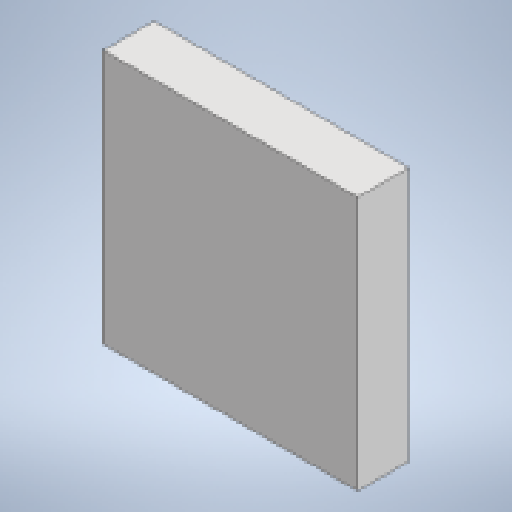
# Autodesk Inventor part: Contrapeso
Saved by Autodesk Inventor 2024 (Build 280153000, 153)
## iProperties
Created: 2024-07-16
Part Number: Contrapeso
Material: Genérico
Document SubType Name: Modeling
Designer: sergi
Density: 1 g/cm^3
Appearance: Valor por defecto
Author: sergi
Autodesk Inventor part; units mm, degrees
ref_plane "YZ Plane" through (0, 0, 0) normal (1, 0, 0) x (0, 1, 0)
ref_plane "XZ Plane" through (0, 0, 0) normal (0, 1, 0) x (-1, 0, 0)
ref_plane "XY Plane" through (0, 0, 0) normal (0, 0, 1) x (1, 0, 0)
sketch "Boceto1" plane through (0, 0, 0) normal (0, 0, 1) x (1, 0, 0)
  line L0 (0, -3) -> (0, -206) projected
  line L1 (0, -3) -> (-3, -3) projected
  line L2 (-3, -206) -> (-3, -3) projected
  line L3 (0, -206) -> (-3, -206) projected
  line L4 (-206, -203) -> (-206, 0) projected
  line L5 (-206, -203) -> (-203, -203) projected
  line L6 (-203, 0) -> (-203, -203) projected
  line L7 (-206, 0) -> (-203, 0) projected
  line L8 (-203, -203) -> (-3, -203)
  line L9 (-3, -203) -> (-3, -3)
  line L10 (-3, -3) -> (-203, -3)
  line L11 (-203, -3) -> (-203, -203)
  line L12 (-103, -203) -> (-103, -163)
  line L13 (-103, -163) -> (-143, -163)
  line L14 (-143, -163) -> (-63, -163)
  line L15 (-63, -163) -> (-63, -203)
  line L16 (-63, -203) -> (-143, -203)
  line L17 (-143, -203) -> (-143, -163)
  line L18 (-147.5, -3) -> (-147.5, -20.5)
  line L19 (-158.5, -20.5) -> (-158.5, -3)
  line L20 (-147.5, -3) -> (-147.5, -20.5)
  line L21 (-158.5, -3) -> (-147.5, -3) projected
  circle A0 centre (-191, -53) radius 2.1 projected
  line L22 (-185.5, -58.5) -> (-203, -58.5) projected
  line L23 (-185.5, -47.5) -> (-185.5, -58.5) projected
  line L24 (-203, -47.5) -> (-185.5, -47.5) projected
  line L25 (-203, -58.5) -> (-203, -47.5) projected
  circle A1 centre (-53, -15) radius 2.1 projected
  line L26 (-58.5, -20.5) -> (-58.5, -3) projected
  line L27 (-47.5, -20.5) -> (-58.5, -20.5) projected
  line L28 (-47.5, -3) -> (-47.5, -20.5) projected
  line L29 (-58.5, -3) -> (-47.5, -3) projected
  circle A2 centre (-15, -53) radius 2.1 projected
  line L30 (-20.5, -47.5) -> (-3, -47.5) projected
  line L31 (-20.5, -58.5) -> (-20.5, -47.5) projected
  line L32 (-3, -58.5) -> (-20.5, -58.5) projected
  line L33 (-3, -47.5) -> (-3, -58.5) projected
  line L34 (-20.5, -147.5) -> (-3, -147.5) projected
  line L35 (-3, -158.5) -> (-20.5, -158.5) projected
  line L36 (-20.5, -158.5) -> (-20.5, -147.5) projected
  line L37 (-47.5, -185.5) -> (-47.5, -203) projected
  line L38 (-58.5, -203) -> (-58.5, -185.5) projected
  line L39 (-58.5, -185.5) -> (-47.5, -185.5) projected
  line L40 (-158.5, -203) -> (-158.5, -185.5) projected
  line L41 (-158.5, -185.5) -> (-147.5, -185.5) projected
  line L42 (-147.5, -185.5) -> (-147.5, -203) projected
  line L43 (-185.5, -158.5) -> (-203, -158.5) projected
  line L44 (-203, -147.5) -> (-185.5, -147.5) projected
  line L45 (-185.5, -147.5) -> (-185.5, -158.5) projected
  line L46 (-158.5, -3) -> (-147.5, -3)
  line L47 (-147.5, -3) -> (-147.5, -20.5)
  line L48 (-158.5, -20.5) -> (-158.5, -3)
  line L49 (-158.5, -3) -> (-147.5, -3)
  line L50 (-147.5, -3) -> (-147.5, -20.5)
  line L51 (-147.5, -20.5) -> (-158.5, -20.5)
  line L52 (-158.5, -20.5) -> (-158.5, -3)
  line L53 (-147.5, -22.5) -> (-160.5, -22.5)
  line L54 (-160.5, -22.5) -> (-160.5, -3)
  line L55 (-160.5, -3) -> (-145.5, -3)
  line L56 (-145.5, -3) -> (-145.5, -22.5)
  line L57 (-145.5, -22.5) -> (-160.5, -22.5)
  line L58 (-160.5, -22.5) -> (-160.5, -3)
  circle A3 centre (-103, -103) radius 47 projected
  line L59 (-47.5, -22.5) -> (-60.5, -22.5)
  line L60 (-60.5, -22.5) -> (-60.5, -3)
  line L61 (-45.5, -3) -> (-45.5, -22.5)
  line L62 (-45.5, -22.5) -> (-60.5, -22.5)
  line L63 (-60.5, -22.5) -> (-60.5, -3)
  line L64 (-183.5, -160.5) -> (-203, -160.5)
  line L65 (-203, -147.5) -> (-185.5, -147.5)
  line L66 (-203, -147.5) -> (-185.5, -147.5)
  line L67 (-185.5, -158.5) -> (-203, -158.5)
  line L68 (-183.5, -160.5) -> (-203, -160.5)
  line L69 (-185.5, -158.5) -> (-203, -158.5)
  line L70 (-185.5, -158.5) -> (-203, -158.5)
  line L71 (-183.5, -147.5) -> (-183.5, -160.5)
  line L72 (-203, -147.5) -> (-185.5, -147.5)
  line L73 (-203, -147.5) -> (-185.5, -147.5)
  line L74 (-185.5, -147.5) -> (-185.5, -158.5)
  line L75 (-183.5, -145.5) -> (-183.5, -160.5)
  line L76 (-203, -145.5) -> (-183.5, -145.5)
  line L77 (-183.5, -47.5) -> (-183.5, -60.5)
  line L78 (-183.5, -45.5) -> (-183.5, -60.5)
  line L79 (-183.5, -60.5) -> (-203, -60.5)
  line L80 (-183.5, -60.5) -> (-203, -60.5)
  line L81 (-203, -45.5) -> (-183.5, -45.5)
  line L82 (-45.5, -183.5) -> (-45.5, -203)
  line L83 (-58.5, -203) -> (-58.5, -185.5)
  line L84 (-58.5, -203) -> (-58.5, -185.5)
  line L85 (-47.5, -185.5) -> (-47.5, -203)
  line L86 (-45.5, -183.5) -> (-45.5, -203)
  line L87 (-47.5, -185.5) -> (-47.5, -203)
  line L88 (-47.5, -185.5) -> (-47.5, -203)
  line L89 (-58.5, -183.5) -> (-45.5, -183.5)
  line L90 (-58.5, -203) -> (-58.5, -185.5)
  line L91 (-58.5, -203) -> (-58.5, -185.5)
  line L92 (-58.5, -185.5) -> (-47.5, -185.5)
  line L93 (-60.5, -183.5) -> (-45.5, -183.5)
  line L94 (-60.5, -203) -> (-60.5, -183.5)
  line L95 (-158.5, -183.5) -> (-145.5, -183.5)
  line L96 (-160.5, -183.5) -> (-145.5, -183.5)
  line L97 (-145.5, -183.5) -> (-145.5, -203)
  line L98 (-145.5, -183.5) -> (-145.5, -203)
  line L99 (-160.5, -203) -> (-160.5, -183.5)
  line L100 (-22.5, -45.5) -> (-3, -45.5)
  line L101 (-3, -58.5) -> (-20.5, -58.5)
  line L102 (-3, -58.5) -> (-20.5, -58.5)
  line L103 (-20.5, -47.5) -> (-3, -47.5)
  line L104 (-22.5, -45.5) -> (-3, -45.5)
  line L105 (-20.5, -47.5) -> (-3, -47.5)
  line L106 (-20.5, -47.5) -> (-3, -47.5)
  line L107 (-22.5, -58.5) -> (-22.5, -45.5)
  line L108 (-3, -58.5) -> (-20.5, -58.5)
  line L109 (-3, -58.5) -> (-20.5, -58.5)
  line L110 (-20.5, -58.5) -> (-20.5, -47.5)
  line L111 (-22.5, -60.5) -> (-22.5, -45.5)
  line L112 (-3, -60.5) -> (-22.5, -60.5)
  line L113 (-22.5, -158.5) -> (-22.5, -145.5)
  line L114 (-22.5, -160.5) -> (-22.5, -145.5)
  line L115 (-22.5, -145.5) -> (-3, -145.5)
  line L116 (-22.5, -145.5) -> (-3, -145.5)
  line L117 (-3, -160.5) -> (-22.5, -160.5)
  line L118 (-145.5, -183.5) -> (-60.5, -183.5)
  point P0 (0, 0)
  point P1 (-3, -203)
  point P2 (-3, -45.5)
  point P3 (-63, -183.5)
  point P4 (-143, -183.5)
  dimension "d3" = 40
  dimension "d4" = 40
  dimension "d5" = 80
  dimension "d6" = 2
  dimension "d7" = 15
  dimension "d8" = 15
  dimension "d11" = 360
  constraints: 172 end point, 10 parallel, 7 perpendicular, 5 horizontal, 1 midpoint, 1 point on line, 1 vertical, 154 other
  measures "d3" distance of L12.start L12.end
  measures "d4" distance of L12.end L13.end
  measures "d5" distance of L15.end L16.end
  measures "d6" distance between parallel lines of L51 L53
  measures "d7" distance of L56.end L57.end
  measures "d8" distance of L61.end L62.end
extrude "Extrusión1" add sketch "Boceto1" against normal blind 40 contours L2 L100 L107 L111 L112 L115 L113 L114 L117 L8 L82 L89 L93 L118 L15 L14 L13 L17 L95 L96 L99 L6 L64 L71 L75 L76 L79 L77 L78 L81 L10 L54 L53 L57 L56 L60 L59 L62 L61 | A3
shell "Vaciado1" thickness 0.8 removed faces 1 at (-103, -69.3333, -40)
